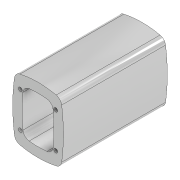
# Autodesk Inventor part: lineaire as deel 1
Saved by Autodesk Inventor 2020.3 (Build 243373000, 373)
## iProperties
Created: 2020-09-16
Part Number: lineaire as deel 1
Material: Aluminum 6061
Document SubType Name: Modeling
Designer: Svend
Density: 2.7 g/cm^3
Appearance: Aluminum - Polished
Author: Svend
Autodesk Inventor part; units mm, degrees
ref_plane "YZ Plane" through (0, 0, 0) normal (1, 0, 0) x (0, 1, 0)
ref_plane "XZ Plane" through (0, 0, 0) normal (0, 1, 0) x (-1, 0, 0)
ref_plane "XY Plane" through (0, 0, 0) normal (0, 0, 1) x (1, 0, 0)
sketch "Sketch1" plane through (0, 0, 0) normal (0, 0, 1) x (1, 0, 0)
  circle A0 centre (-57, 57.5) radius 3
  circle A1 centre (57, 57.5) radius 3
  circle A2 centre (-57, -57.5) radius 3
  circle A3 centre (57, -57.5) radius 3
  line L0 (-57, -57.5) -> (57, 57.5) construction
  line L1 (-67.5, 67.5) -> (67.5, 67.5) construction
  line L2 (67.5, 67.5) -> (67.5, -67.5) construction
  line L3 (67.5, -67.5) -> (-67.5, -67.5) construction
  line L4 (-67.5, -67.5) -> (-67.5, 67.5) construction
  line L5 (-67.5, 67.5) -> (67.5, -67.5) construction
  line L6 (67.5, 67.5) -> (-67.5, -67.5) construction
  circle A4 centre (-37.5, 37.5) radius 4
  circle A5 centre (-37.5, -37.5) radius 4
  circle A6 centre (37.5, -37.5) radius 4
  circle A7 centre (37.5, 37.5) radius 4
  arc A8 (-48.5, 62.5) -> (-48.5, -62.5) centre (326.325, 0) ccw
  line L7 (0, 67.5) -> (0, -67.5) construction
  line L8 (67.5, -67.5) -> (67.5, 67.5) construction
  arc A9 (48.5, -62.5) -> (48.5, 62.5) centre (-326.325, 0) ccw
  arc A10 (48.5, 62.5) -> (-48.5, 62.5) centre (0, -110.8429) ccw
  line L9 (-67.5, 0) -> (53.675, 0) construction
  arc A11 (-48.5, -62.5) -> (48.5, -62.5) centre (0, 110.8429) ccw
  arc A12 (-30.7003, 46.1842) -> (-30.7003, -46.1842) centre (326.325, 0) ccw
  arc A13 (-30.7003, -46.1842) -> (30.7003, -46.1842) centre (0, 110.8429) ccw
  arc A14 (30.7003, -46.1842) -> (30.7003, 46.1842) centre (-326.325, 0) ccw
  arc A15 (30.7003, 46.1842) -> (-30.7003, 46.1842) centre (0, -110.8429) ccw
  point P0 (0, 0)
  point P1 (0, 0)
  point P2 (-53.675, 0)
  point P3 (0, 0)
  dimension "d0" = 114
  dimension "d1" = 115
  dimension "d2" = 6
  dimension "d3" = 135
  dimension "d4" = 135
  dimension "d5" = 8
  dimension "d9" = 360
  dimension "d29" = 75
  dimension "d30" = 125
  dimension "d31" = 97
  dimension "d32" = 180
  dimension "d33" = 380
  dimension "d34" = 20
  constraints: 20 end point, 17 point on circle, 16 centre point, 7 midpoint, 5 symmetric about line, 3 equal radius, 3 horizontal alignment, 2 horizontal, 2 parallel, 2 vertical alignment, 1 coincident, 1 perpendicular, 1 point on line, 14 other
  measures "d0" distance of L0.end A0.centre
  measures "d1" distance of A3.centre L0.end
  measures "d2" diameter of A1
  measures "d3" distance of L2.end L3.end
  measures "d4" distance of L1.end L2.end
  measures "d5" diameter of A4
  measures "d29" distance of A4.centre A7.centre
  measures "d30" distance of A8.end A8.start
  measures "d31" distance of A9.end A8.start
  measures "d32" radius of A10
  measures "d33" radius of A8
  measures "d34" radial gap between concentric circles of A10 A15
extrude "Extrusion1" add sketch "Sketch1" along normal mid plane 220 contours A10 A9 A11 A8
fillet "Fillet2" radius 15 8 edges at (48.5, 62.5, 0) (-48.5, 62.5, 0) (-48.5, -62.5, 0) (48.5, -62.5, 0) (-30.7003, 46.1842, 0) (30.7003, 46.1842, 0) (30.7003, -46.1842, 0) (-30.7003, -46.1842, 0)
body "Solid1"
